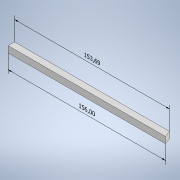
# Autodesk Inventor part: Support1
Saved by Autodesk Inventor 2020.1 (Build 241239000, 239)
## iProperties
Created: 2019-12-12
Part Number: Support1
Material: Generic
Document SubType Name: Modeling
Designer: super
Density: 1 g/cm^3
Appearance: Default
Author: super
Autodesk Inventor part; units mm, degrees
ref_plane "YZ Plane" through (0, 0, 0) normal (1, 0, 0) x (0, 1, 0)
ref_plane "XZ Plane" through (0, 0, 0) normal (0, 1, 0) x (-1, 0, 0)
ref_plane "XY Plane" through (0, 0, 0) normal (0, 0, 1) x (1, 0, 0)
sketch "Sketch1" plane through (0, 0, 0) normal (0, 1, 0) x (-1, 0, 0)
  line L0 (0, 0) -> (-156, 0)
  line L1 (0, -6.35) -> (0, 0)
  line L2 (-156, 0) -> (-153.6888, -6.35)
  line L3 (-156, 0) -> (-149.2425, 0) construction
  line L4 (0, -6.35) -> (-153.6888, -6.35)
  dimension "d0" = 156
  dimension "d2" = 70
  constraints: 10 end point, 3 horizontal, 1 equal length, 1 perpendicular
  measures "d0" distance of L0.start L0.end
  measures "d2" angle of L2 L3
extrude "Extrusion1" add sketch "Sketch1" along normal blind 6.35
body "Solid1"
